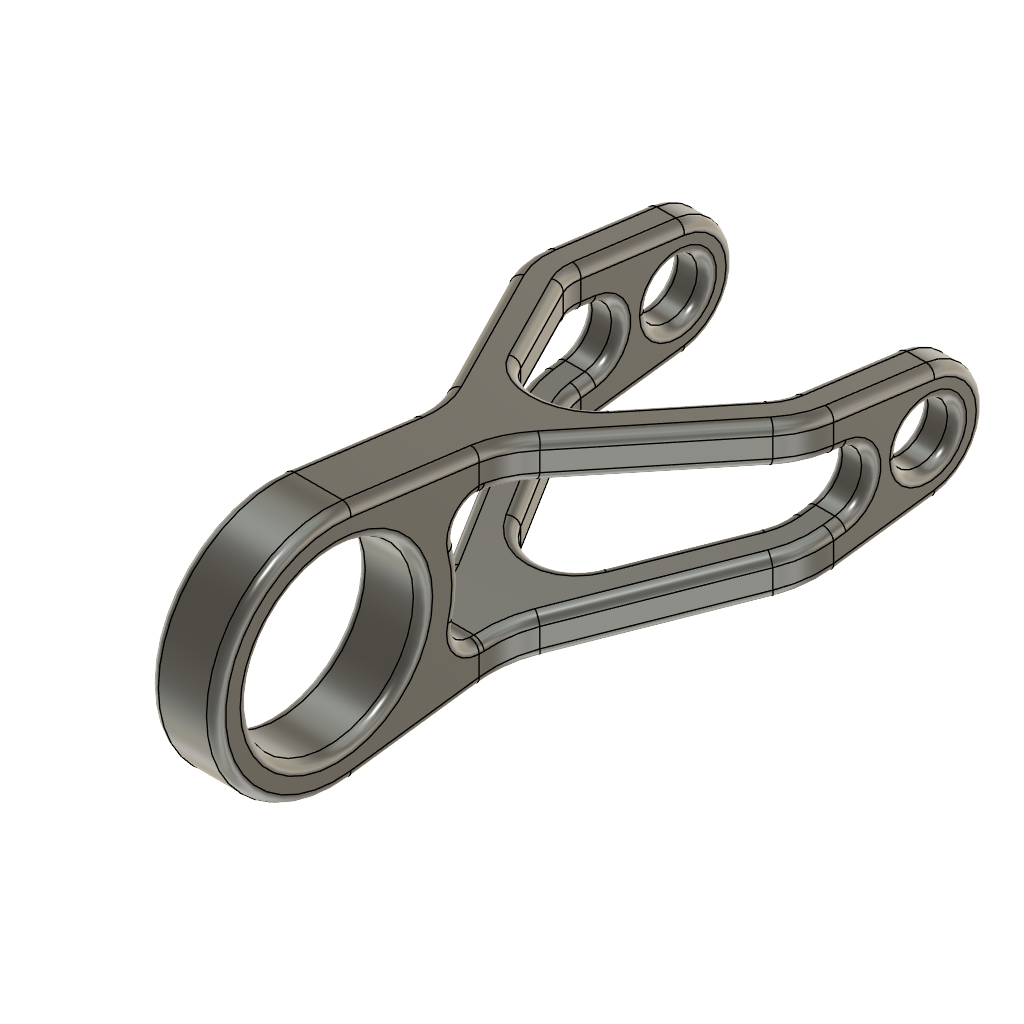
fusion exercise 5 (Autodesk Fusion 360 design; units mm, degrees)
part number: 2026-09-22-16-55-20-294
Autodesk Fusion 360 part; units mm, degrees
sketch "Sketch1" plane through (0, 0, 0) normal (1, 0, 0) x (0, 1, 0)
  line L0 (0, 0) -> (100, 0) construction
  circle A0 centre (0, 0) radius 18
  circle A1 centre (100, 0) radius 6
  line L1 (3.25, 24.7878) -> (101.56, 11.8982)
  line L2 (3.25, -24.7878) -> (101.56, -11.8982)
  arc A2 (101.56, -11.8982) -> (101.56, 11.8982) centre (100, 0) ccw
  arc A3 (3.25, 24.7878) -> (3.25, -24.7878) centre (0, 0) ccw
  arc A4 (25.078, -6.8626) -> (25.078, 6.8626) centre (0, 0) ccw
  line L3 (30.5507, -13.1399) -> (82.6411, -6.3102)
  arc A5 (30.5507, 13.1399) -> (25.078, 6.8626) centre (29.9007, 8.1824) ccw
  arc A6 (25.078, -6.8626) -> (30.5507, -13.1399) centre (29.9007, -8.1824) ccw
  line L4 (94, 0) -> (94, 0.0041)
  arc A7 (82.6411, -6.3102) -> (82.6411, 6.3102) centre (81.8137, 0) ccw
  line L5 (30.5507, 13.1399) -> (82.6411, 6.3102)
  dimension "d1" = 24
  dimension "d2" = 12
  dimension "d3" = 50
  dimension "d4" = 36
  dimension "d5" = 100
  dimension "d6" = 26
  dimension "d9" = 5
  dimension "d10" = 5
  constraint coincident L0.start A0.centre
  constraint horizontal L0
  constraint coincident L0.end A1.centre
  constraint concentric A1 A2
  constraint tangent L1 A3
  constraint tangent L1 A2
  constraint symmetric L0 L1.start L2.start
  constraint symmetric L0 L1.end L2.end
  constraint tangent A5 L5
  constraint tangent A4 A5
  constraint tangent A4 A6
  constraint tangent L3 A6
  constraint coincident A1 L4.start
  constraint coincident L0 L4.start
  constraint perpendicular L0 L4
  constraint tangent L3 A7
  constraint coincident A1 L4.end
  measures "d1" diameter of A2
  measures "d2" diameter of A1
  measures "d3" diameter of A3
  measures "d4" diameter of A0
  measures "d5" distance of L0.start L0.end
  measures "d6" radius of A4
  measures "d9" radius of A5
  measures "d10" radius of A6
extrude "Extrude1" add sketch "Sketch1" along normal mid plane 60
ref_plane "WorkPlane1" through (0, 0, 60) normal (0, 0, 1) x (1, 0, 0)
sketch "Sketch2" plane through (0, 0, 60) normal (0, 0, 1) x (1, 0, 0)
  line L0 (-30, 3.25) -> (-30, -25)
  line L1 (-30, -25) -> (30, -25)
  line L2 (30, -25) -> (30, 3.25)
  line L3 (30, 3.25) -> (30, 101.56)
  line L4 (30, 101.56) -> (30, 112)
  line L5 (-30, 112) -> (30, 112)
  line L6 (-30, 112) -> (-30, 101.56)
  line L7 (-30, 101.56) -> (-30, 3.25)
  line L8 (0, -25) -> (0, 112)
  line L9 (-7, -25) -> (-7, 29.6599)
  line L10 (-9.6619, 39.6293) -> (-27.3381, 70.3707)
  line L11 (-30, 80.3401) -> (-30, 112)
  line L12 (30, 106) -> (30, 94) construction
  line L13 (30, 100) -> (-30, 100) construction
  line L14 (-30, 112) -> (-22, 112)
  line L15 (-22, 112) -> (-22, 79.8061)
  line L16 (-20.6691, 74.8214) -> (-8.6691, 53.9518)
  line L17 (20.6691, 74.8214) -> (8.6691, 53.9518)
  line L18 (9.6619, 39.6293) -> (27.3381, 70.3707)
  line L19 (7, -25) -> (7, 29.6599)
  line L20 (22, 112) -> (22, 79.8061)
  line L21 (30, 80.3401) -> (30, 112)
  line L22 (30, 112) -> (22, 112)
  arc A0 (-7, 29.6599) -> (-9.6619, 39.6293) centre (-27, 29.6599) ccw
  arc A1 (9.6619, 39.6293) -> (7, 29.6599) centre (27, 29.6599) ccw
  arc A2 (-30, 80.3401) -> (-27.3381, 70.3707) centre (-10, 80.3401) ccw
  arc A3 (27.3381, 70.3707) -> (30, 80.3401) centre (10, 80.3401) ccw
  arc A4 (20.6691, 74.8214) -> (22, 79.8061) centre (12, 79.8061) ccw
  arc A5 (-22, 79.8061) -> (-20.6691, 74.8214) centre (-12, 79.8061) ccw
  arc A6 (-8.6691, 53.9518) -> (8.6691, 53.9518) centre (0, 58.9365) ccw
  point P0 (-7, 35)
  point P1 (-30, 75)
  dimension "d16" = 14
  dimension "d17" = 35
  dimension "d18" = 75
  dimension "d20" = 12
  dimension "d21" = 8
  dimension "d22" = 8
  dimension "d23" = 20
  dimension "d24" = 20
  dimension "d25" = 20
  dimension "d26" = 20
  dimension "d27" = 10
  dimension "d28" = 10
  dimension "d29" = 10
  constraint midpoint L1 L8.start
  constraint midpoint L5 L8.end
  constraint coincident L1 L9.start
  constraint perpendicular L1 L9
  constraint perpendicular L5 L11
  constraint coincident L6.end L11
  constraint midpoint L12 L13.start
  constraint coincident L11 L13.end
  constraint perpendicular L6 L14
  constraint perpendicular L13 L15
  constraint parallel L10 L16
  constraint symmetric L8 L9.start L19.start
  constraint symmetric L8 L5.start L4.end
  constraint symmetric L8 L14.end L20.start
  constraint coincident P0 L9
  constraint coincident P0 L10
  constraint tangent L9 A0
  constraint tangent L10 A0
  constraint tangent L18 A1
  constraint tangent L19 A1
  constraint coincident P1 L10
  constraint coincident P1 L11
  constraint tangent L10 A2
  constraint tangent L11 A2
  constraint tangent L18 A3
  constraint tangent L21 A3
  constraint tangent L17 A4
  constraint tangent L20 A4
  constraint tangent L15 A5
  constraint tangent L16 A5
  constraint tangent L16 A6
  constraint tangent L17 A6
  measures "d17" vertical distance of origin P0
  measures "d18" vertical distance of P1 origin
  measures "d20" distance of L5.start L13.end
  measures "d21" distance of L5.start L14.end
  measures "d22" distance of L10 L16
  measures "d23" radius of A0
  measures "d24" radius of A1
  measures "d25" radius of A2
  measures "d26" radius of A3
  measures "d27" radius of A4
  measures "d28" radius of A5
  measures "d29" radius of A6
extrude "Extrude2" cut sketch "Sketch2" against normal blind 100 contours L0 L1 L7 L9 L10 A0 A2 | L1 L2 L3 L18 L19 A1 A3 | L5 L8 L15 L16 A5 A6 | L5 L8 L17 L20 A4 A6
fillet "Fillet1" radius 2 94 edges at (18.5, 55, 18.0028) (29.3231, 75.1807, 15.3568) (30, 90.95, 13.2893) (30, 112, 0) (30, 90.95, -13.2893) (29.3231, 75.1807, -15.3568) (18.5, 55, -18.0028) (7.6769, 34.8193, -20.6487) (7, 16.455, -23.0565) (7, -25, 0) (7, 16.455, 23.0565) (7.6769, 34.8193, 20.6487) (-7, -25, 0) (-7, 16.455, -23.0565) (-7.6769, 34.8193, -20.6487) (-18.5, 55, -18.0028) (-29.3231, 75.1807, -15.3568) (-30, 90.95, -13.2893) (-30, 112, 0) (-30, 90.95, 13.2893) (-29.3231, 75.1807, 15.3568) (-18.5, 55, 18.0028) (-7.6769, 34.8193, 20.6487) (-7, 16.455, 23.0565) (-29.3231, 75.1807, 7.2884) (-30, 81.4906, 6.4611) (-30, 88.178, 0) (-30, 81.4906, -6.4611) (-29.3231, 75.1807, -7.2884) (-18.5, 55, -9.9343) (-7.7966, 35.2484, -12.524) (-7.0049, 30.1024, -13.1783) (-7, 25.8539, -11.119) (-7, 26, 0) (-7, 25.8539, 11.119) (-7.0049, 30.1024, 13.1783) (-7.7966, 35.2484, 12.524) (-18.5, 55, 9.9343) (-21.6615, 77.2264, 15.0886) (-22, 90.683, 13.3243) (-22, 112, 0) (-22, 90.683, -13.3243) (-21.6615, 77.2264, -15.0886) (-14.6691, 64.3866, -16.7721) (0, 48.9365, -18.7978) (14.6691, 64.3866, -16.7721) (21.6615, 77.2264, -15.0886) (22, 90.683, -13.3243) (22, 112, 0) (22, 90.683, 13.3243) (21.6615, 77.2264, 15.0886) (14.6691, 64.3866, 16.7721) (0, 48.9365, 18.7978) (-14.6691, 64.3866, 16.7721) (29.3231, 75.1807, -7.2884) (30, 81.4906, -6.4611) (30, 88.178, 0) (30, 81.4906, 6.4611) (29.3231, 75.1807, 7.2884) (18.5, 55, 9.9343) (7.7966, 35.2484, 12.524) (7.0049, 30.1024, 13.1783) (7, 25.8539, 11.119) (7, 26, 0) (7, 25.8539, -11.119) (7.0049, 30.1024, -13.1783) (7.7966, 35.2484, -12.524) (18.5, 55, -9.9343) (7, -16.7819, -6.5091) (-7, -16.7819, 6.5091) (-30, 105.5947, 2.1678) (-30, 94, 0.002) (22, 105.5932, -2.1716) (22, 94, 0.002) (-22, 105.5947, 2.1678) (-22, 94, 0.002) (30, 105.5932, -2.1716) (30, 94, 0.002) (-22, 81.2236, -6.4961) (-22, 88.178, 0) (-22, 81.2236, 6.4961) (-21.6615, 77.2264, 7.0201) (-14.6691, 64.3866, 8.7036) (0, 48.9365, 10.7293) (14.6691, 64.3866, 8.7036) (21.6615, 77.2264, 7.0201) (22, 81.2236, 6.4961) (22, 88.178, 0) (22, 81.2236, -6.4961) (21.6615, 77.2264, -7.0201) (14.6691, 64.3866, -8.7036) (0, 48.9365, -10.7293) (-14.6691, 64.3866, -8.7036) (-21.6615, 77.2264, -7.0201)
